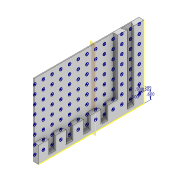
# Autodesk Inventor part: Lift receiver left side actobtics
Saved by Autodesk Inventor 2020 (Build 240168000, 168)
## iProperties
Created: 2019-11-10
Part Number: Lift receiver left side actobtics
Material: Generic
Document SubType Name: Modeling
Designer: ball
Density: 1 g/cm^3
Appearance: Default
Author: ball
Autodesk Inventor part; units mm, degrees
ref_plane "YZ Plane" through (0, 0, 0) normal (1, 0, 0) x (0, 1, 0)
ref_plane "XZ Plane" through (0, 0, 0) normal (0, 1, 0) x (-1, 0, 0)
ref_plane "XY Plane" through (0, 0, 0) normal (0, 0, 1) x (1, 0, 0)
sketch "Sketch1" plane through (0, 0, 0) normal (0, 1, 0) x (-1, 0, 0)
  line L0 (7.366, 6.1452) -> (7.366, -23.8548)
  line L1 (7.366, -23.8548) -> (0, -23.8548)
  line L2 (6.096, -8.0476) -> (6.096, -9.0212)
  line L3 (0, 0.4868) -> (0, 3.5348)
  line L4 (6.096, 3.5348) -> (6.096, -8.0476)
  line L5 (0, -9.0212) -> (0, -11.8152)
  line L6 (6.096, -12.0692) -> (6.096, -9.0212)
  line L7 (6.096, 3.5348) -> (0, 0.4868)
  line L8 (6.096, -12.0692) -> (0, -9.0212)
  line L9 (0, -23.8548) -> (0, -9.0212)
  line L10 (0, 0.4868) -> (0, 16.3788)
  line L11 (6.096, 13.3308) -> (6.096, 16.3788)
  line L12 (6.096, 13.3308) -> (0, 16.3788)
  line L13 (6.096, 28.9348) -> (6.096, 17.3524)
  line L14 (6.096, 28.9348) -> (0, 25.8868)
  line L15 (6.096, 17.3524) -> (6.096, 16.3788)
  line L16 (6.096, 38.7308) -> (6.096, 41.7788)
  line L17 (6.096, 38.7308) -> (0, 41.7788)
  line L18 (6.096, 54.3348) -> (6.096, 42.7524)
  line L19 (6.096, 54.3348) -> (0, 51.2868)
  line L20 (6.096, 42.7524) -> (6.096, 41.7788)
  line L21 (6.096, 64.1308) -> (6.096, 67.1788)
  line L22 (6.096, 64.1308) -> (0, 67.1788)
  line L23 (6.096, 79.7348) -> (6.096, 68.1524)
  line L24 (6.096, 79.7348) -> (0, 76.6868)
  line L25 (6.096, 68.1524) -> (6.096, 67.1788)
  line L26 (7.366, 6.1452) -> (7.366, 91.622)
  line L27 (7.366, 91.622) -> (0, 91.622)
  line L28 (0, 25.8868) -> (0, 41.7788)
  line L29 (0, 51.2868) -> (0, 67.1788)
  line L30 (0, 76.6868) -> (0, 91.622)
  line L31 (6.096, -4.2672) -> (4.0009, -4.2672) construction
  point P0 (0, 0)
  dimension "d0" = 7.366
  dimension "d8" = 9.508
  dimension "d10" = 3.048
  dimension "d11" = 3.048
  dimension "d12" = 6.096
  dimension "d17" = 25.4
  dimension "d24" = 11.7856
  dimension "d67" = 115.4768
  dimension "d70" = 23.8548
  dimension "d71" = 4.754
  constraints: 64 end point, 5 vertical, 4 parallel, 3 point on line, 2 horizontal, 33 other
  measures "d0" distance of L0.end L1.end
  measures "d8" distance of L5.start L3.start
  measures "d10" vertical distance of L4.start L3.start
  measures "d11" vertical distance of L6.start L5.start
  measures "d12" distance from line of L9 L6.start
  measures "d17" distance of L2.end L11.end
  measures "d24" distance from line of L1 L6.start
  measures "d67" distance between parallel lines of L1 L27
  measures "d70" distance from line of L1 point (0, 0)
  measures "d71" vertical distance of L31.start L3.start
extrude "MultipleTeeth" add sketch "Sketch1" along normal blind 19.05
sketch "Sketch2" plane through (0, 0, 0) normal (0, -1, 0) x (1, 0, 0)
  line L0 (0, 0.4868) -> (-6.096, 3.5348) construction
  line L1 (-6.096, 3.5348) -> (-6.096, -12.0692) construction
  line L2 (-6.096, -12.0692) -> (0, -9.0212) construction
  line L3 (0, 16.3788) -> (0, 0.4868) projected
  line L4 (0, 0.4868) -> (-6.096, 3.5348)
  line L5 (-6.096, -12.0692) -> (0, -9.0212) projected
  line L6 (-6.096, 3.5348) -> (-6.096, -12.0692) projected
  line L7 (-6.096, -12.0692) -> (-6.096, 3.5348)
  line L8 (0, -9.0212) -> (-6.096, -12.0692)
  line L9 (-7.366, -23.8548) -> (-7.366, 91.622) projected
  line L10 (-7.366, -59.508) -> (-7.366, -32.8548)
  line L11 (-7.366, -23.8548) -> (0, -23.8548)
  line L12 (-7.366, 91.622) -> (0, 91.622) projected
  line L13 (-7.366, -55.8503) -> (-7.366, -40.458) construction
  line L14 (0, -43.0234) -> (0, -59.508) construction
  line L15 (-6.096, -62.0648) -> (0, -62.0648) construction
  line L16 (0, -32.8548) -> (0, -37.6258)
  line L17 (0, -49.9828) -> (0, -62.0648)
  line L18 (0, -62.0648) -> (0, -59.508)
  line L19 (0, -32.8548) -> (-7.366, -32.8548) construction
  line L20 (0, -51.9048) -> (-7.366, -51.9048) construction
  line L21 (0, -42.3798) -> (-7.366, -42.3798) construction
  line L22 (-6.096, -12.0692) -> (-6.096, -62.0648) construction
  line L23 (0, -37.6258) -> (-6.096, -34.5778)
  line L24 (-6.096, -50.1818) -> (-6.096, -34.5778)
  line L25 (0, -47.1338) -> (-6.096, -50.1818)
  line L26 (0, -9.0212) -> (0, -23.8548) projected
  line L27 (0, -23.8548) -> (0, -32.8548)
  line L28 (-7.366, -32.8548) -> (-7.366, -23.8548)
  line L29 (0, -49.9828) -> (0, -47.1338)
  line L30 (0, -62.0648) -> (-7.366, -62.0648)
  line L31 (-7.366, -62.0648) -> (-7.366, -59.508)
  point P0 (0, 0)
  dimension "d25" = 115.4768
  dimension "d33" = 9
  dimension "d34" = 19.05
  dimension "d36" = 9.525
  dimension "d38" = 10.16
  constraints: 46 end point, 4 parallel, 4 perpendicular, 4 point on line, 3 collinear, 2 horizontal, 2 vertical
  measures "d25" distance between parallel lines of L12 L11
  measures "d33" distance of L16.start L11.end
  measures "d34" distance between parallel lines of L20 L19
  measures "d36" distance between parallel lines of L21 L19
  measures "d38" distance between parallel lines of L15 L20
extrude "LongTooth" add sketch "Sketch2" against normal blind 100.2792
sketch "Sketch3" plane through (0, 19.05, 0) normal (0, 1, 0) x (1, 0, 0)
  line L0 (-6.096, -3.5348) -> (-6.096, 12.0692) construction
  line L1 (0, 23.8548) -> (-7.366, 23.8548) projected
  line L2 (-7.366, -91.622) -> (0, -91.622) projected
  line L3 (-7.366, 23.8548) -> (-6.096, 23.8548)
  line L4 (-6.096, 23.8548) -> (-6.096, -91.622)
  line L5 (-6.096, -91.622) -> (-7.366, -91.622)
  line L6 (-7.366, -91.622) -> (-7.366, 23.8548)
  point P0 (0, 0)
  constraints: 8 end point, 2 parallel, 1 horizontal, 1 perpendicular, 1 point on line
extrude "ThinPlate" add sketch "Sketch3" along normal up to surface (81.2292 mm away)
sketch "Sketch4" plane through (0, 0, 0) normal (0, -1, 0) x (1, 0, 0)
  line L0 (-6.096, 91.622) -> (0, 91.622) projected
  line L1 (-7.366, 91.622) -> (-7.366, -62.0648) projected
  line L2 (0, 91.622) -> (-7.366, 91.622)
  line L3 (-7.366, 91.622) -> (-7.366, -62.0648)
  line L4 (-7.366, -62.0648) -> (0, -62.0648)
  line L5 (0, -62.0648) -> (0, 91.622)
  point P0 (0, 0)
  constraints: 8 end point, 2 parallel, 1 horizontal, 1 perpendicular
extrude "Extrusion4" add sketch "Sketch4" along normal blind 5.08
ref_plane "Work Plane1" through (-15.892, 0, 8.4328) normal (0, 0, 1) x (0, 1, 0)
sketch "Sketch6" plane through (0, 19.05, 16.3788) normal (1, 0, 0) x (0, 0, -1)
  circle A0 centre (71.4586, -8.89) radius 1.9304
  line L0 (78.4436, 81.2292) -> (78.4436, -24.13) projected
  line L1 (78.4436, -24.13) -> (-75.2432, -24.13) projected
  circle A1 centre (58.7586, -8.89) radius 1.9304
  circle A2 centre (46.0586, -8.89) radius 1.9304
  circle A3 centre (71.4586, 3.81) radius 1.9304
  circle A4 centre (58.7586, 3.81) radius 1.9304
  circle A5 centre (46.0586, 3.81) radius 1.9304
  circle A6 centre (71.4586, 16.51) radius 1.9304
  circle A7 centre (58.7586, 16.51) radius 1.9304
  circle A8 centre (46.0586, 16.51) radius 1.9304
  circle A9 centre (71.4586, 29.21) radius 1.9304
  circle A10 centre (58.7586, 29.21) radius 1.9304
  circle A11 centre (46.0586, 29.21) radius 1.9304
  circle A12 centre (71.4586, 41.91) radius 1.9304
  circle A13 centre (58.7586, 41.91) radius 1.9304
  circle A14 centre (46.0586, 41.91) radius 1.9304
  circle A15 centre (71.4586, 54.61) radius 1.9304
  circle A16 centre (58.7586, 54.61) radius 1.9304
  circle A17 centre (46.0586, 54.61) radius 1.9304
  circle A18 centre (71.4586, 67.31) radius 1.9304
  circle A19 centre (58.7586, 67.31) radius 1.9304
  circle A20 centre (46.0586, 67.31) radius 1.9304
  circle A21 centre (71.4586, 80.01) radius 1.9304
  circle A22 centre (58.7586, 80.01) radius 1.9304
  circle A23 centre (46.0586, 80.01) radius 1.9304
  circle A24 centre (33.3586, -8.89) radius 1.9304
  circle A25 centre (33.3586, 3.81) radius 1.9304
  circle A26 centre (33.3586, 16.51) radius 1.9304
  circle A27 centre (33.3586, 29.21) radius 1.9304
  circle A28 centre (33.3586, 41.91) radius 1.9304
  circle A29 centre (33.3586, 54.61) radius 1.9304
  circle A30 centre (33.3586, 67.31) radius 1.9304
  circle A31 centre (33.3586, 80.01) radius 1.9304
  circle A32 centre (20.6586, -8.89) radius 1.9304
  circle A33 centre (20.6586, 3.81) radius 1.9304
  circle A34 centre (20.6586, 16.51) radius 1.9304
  circle A35 centre (20.6586, 29.21) radius 1.9304
  circle A36 centre (20.6586, 41.91) radius 1.9304
  circle A37 centre (20.6586, 54.61) radius 1.9304
  circle A38 centre (20.6586, 67.31) radius 1.9304
  circle A39 centre (20.6586, 80.01) radius 1.9304
  circle A40 centre (7.9586, -8.89) radius 1.9304
  circle A41 centre (7.9586, 3.81) radius 1.9304
  circle A42 centre (7.9586, 16.51) radius 1.9304
  circle A43 centre (7.9586, 29.21) radius 1.9304
  circle A44 centre (7.9586, 41.91) radius 1.9304
  circle A45 centre (7.9586, 54.61) radius 1.9304
  circle A46 centre (7.9586, 67.31) radius 1.9304
  circle A47 centre (7.9586, 80.01) radius 1.9304
  circle A48 centre (-4.7414, -8.89) radius 1.9304
  circle A49 centre (-4.7414, 3.81) radius 1.9304
  circle A50 centre (-4.7414, 16.51) radius 1.9304
  circle A51 centre (-4.7414, 29.21) radius 1.9304
  circle A52 centre (-4.7414, 41.91) radius 1.9304
  circle A53 centre (-4.7414, 54.61) radius 1.9304
  circle A54 centre (-4.7414, 67.31) radius 1.9304
  circle A55 centre (-4.7414, 80.01) radius 1.9304
  circle A56 centre (-17.4414, -8.89) radius 1.9304
  circle A57 centre (-17.4414, 3.81) radius 1.9304
  circle A58 centre (-17.4414, 16.51) radius 1.9304
  circle A59 centre (-17.4414, 29.21) radius 1.9304
  circle A60 centre (-17.4414, 41.91) radius 1.9304
  circle A61 centre (-17.4414, 54.61) radius 1.9304
  circle A62 centre (-17.4414, 67.31) radius 1.9304
  circle A63 centre (-17.4414, 80.01) radius 1.9304
  circle A64 centre (-30.1414, -8.89) radius 1.9304
  circle A65 centre (-30.1414, 3.81) radius 1.9304
  circle A66 centre (-30.1414, 16.51) radius 1.9304
  circle A67 centre (-30.1414, 29.21) radius 1.9304
  circle A68 centre (-30.1414, 41.91) radius 1.9304
  circle A69 centre (-30.1414, 54.61) radius 1.9304
  circle A70 centre (-30.1414, 67.31) radius 1.9304
  circle A71 centre (-30.1414, 80.01) radius 1.9304
  circle A72 centre (-42.8414, -8.89) radius 1.9304
  circle A73 centre (-42.8414, 3.81) radius 1.9304
  circle A74 centre (-42.8414, 16.51) radius 1.9304
  circle A75 centre (-42.8414, 29.21) radius 1.9304
  circle A76 centre (-42.8414, 41.91) radius 1.9304
  circle A77 centre (-42.8414, 54.61) radius 1.9304
  circle A78 centre (-42.8414, 67.31) radius 1.9304
  circle A79 centre (-42.8414, 80.01) radius 1.9304
  circle A80 centre (-55.5414, -8.89) radius 1.9304
  circle A81 centre (-55.5414, 3.81) radius 1.9304
  circle A82 centre (-55.5414, 16.51) radius 1.9304
  circle A83 centre (-55.5414, 29.21) radius 1.9304
  circle A84 centre (-55.5414, 41.91) radius 1.9304
  circle A85 centre (-55.5414, 54.61) radius 1.9304
  circle A86 centre (-55.5414, 67.31) radius 1.9304
  circle A87 centre (-55.5414, 80.01) radius 1.9304
  circle A88 centre (-68.2414, -8.89) radius 1.9304
  circle A89 centre (-68.2414, 3.81) radius 1.9304
  circle A90 centre (-68.2414, 16.51) radius 1.9304
  circle A91 centre (-68.2414, 29.21) radius 1.9304
  circle A92 centre (-68.2414, 41.91) radius 1.9304
  circle A93 centre (-68.2414, 54.61) radius 1.9304
  circle A94 centre (-68.2414, 67.31) radius 1.9304
  circle A95 centre (-68.2414, 80.01) radius 1.9304
  circle A96 centre (-80.9414, -8.89) radius 1.9304
  circle A97 centre (-80.9414, 3.81) radius 1.9304
  circle A98 centre (-80.9414, 16.51) radius 1.9304
  circle A99 centre (-80.9414, 29.21) radius 1.9304
  circle A100 centre (-80.9414, 41.91) radius 1.9304
  circle A101 centre (-80.9414, 54.61) radius 1.9304
  circle A102 centre (-80.9414, 67.31) radius 1.9304
  circle A103 centre (-80.9414, 80.01) radius 1.9304
  point P0 (16.3788, -19.05)
  dimension "d56" = 3.8608
  dimension "d57" = 6.985
  dimension "d58" = 15.24
  dimension "d61" = 12.7
  dimension "d64" = 12.7
  constraints: 104 centre point, 1 horizontal, 1 vertical, 206 other
  measures "d56" diameter of A0
  measures "d57" distance from line of L0 A0.centre
  measures "d58" distance from line of L1 A0.centre
  measures "d61" distance of A0.centre A1.centre
  measures "d64" distance of A0.centre A3.centre
equation "\"d11\" = d10"
equation "\"d71\" = 0.5 * d8"
equation "\"d36\" = 0.5 * d34"
body "Solid1"
